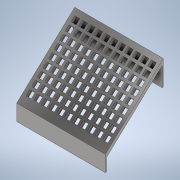
# Autodesk Inventor part: Rejilla_8x8mm
Saved by Autodesk Inventor 2021 (Build 250183000, 183)
## iProperties
Created: 2021-06-27
Part Number: Rejilla_8x8mm
Material: Acero inoxidable
Document SubType Name: Modeling
Designer: artur
Density: 8 g/cm^3
Appearance: Acero - Pulido
Mass: 548.788 g
Surface Area: 547.573 cm^2
Volume: 68.5985 cm^3
Author: artur
Autodesk Inventor part; units mm, degrees
ref_plane "YZ Plane" through (0, 0, 0) normal (1, 0, 0) x (0, 1, 0)
ref_plane "XZ Plane" through (0, 0, 0) normal (0, 1, 0) x (-1, 0, 0)
ref_plane "XY Plane" through (0, 0, 0) normal (0, 0, 1) x (1, 0, 0)
sketch "Boceto7" plane through (-46.053, -27.9809, 0) normal (0, 0, 1) x (1, 0, 0)
  line L0 (118.929, 0) -> (171.1141, 0) construction
  line L1 (-1.0005, -0.9307) -> (-79.0081, -0.9307) construction
  line L2 (-1.0005, -0.9307) -> (89.9995, 83.721)
  line L3 (-1.0005, -0.9307) -> (-1.0005, -25.8991)
  line L4 (-1.0005, -25.8991) -> (0.9995, -25.8991)
  line L5 (0.9995, -25.8991) -> (0.9995, -5.8991)
  line L6 (80.5422, 57.5078) -> (86.2007, 57.5078)
  line L7 (89.9995, 83.721) -> (89.9995, 45.0316)
  line L8 (89.9995, 45.0316) -> (87.9995, 45.0316)
  line L9 (87.9995, 45.0316) -> (87.9995, 75.0316)
  line L10 (0.9995, -5.8991) -> (87.9995, 75.0316)
  dimension "d92" = 137.07
  dimension "d89" = 2
  dimension "d88" = 5
  dimension "d87" = 30
  dimension "d85" = 2
  dimension "d91" = 5
  dimension "d90" = 20
  dimension "d124" = 89
  constraints: 22 end point, 4 horizontal, 2 perpendicular, 2 vertical
  measures "d92" angle of L1 L2
  measures "d89" distance between parallel lines of L5 L3
  measures "d88" distance from line of L2 L9.end
  measures "d87" distance of L8.end L9.end
  measures "d85" distance between parallel lines of L7 L9
  measures "d91" distance from line of L2 L5.end
  measures "d90" distance of L4.end L5.end
  measures "d124" distance between parallel lines of L3 L9
extrude "Extrusión5" add sketch "Boceto7" along normal blind 139
sketch "Boceto8" plane through (-47.0535, -28.9116, 0) normal (-0.6811, 0.7322, 0) x (0, 0, 1)
  line L0 (6, 108.2856) -> (14, 108.2856)
  line L1 (14, 108.2856) -> (14, 116.2856)
  line L2 (14, 116.2856) -> (6, 116.2856)
  line L3 (6, 116.2856) -> (6, 108.2856)
  line L4 (0, 124.2856) -> (139, 124.2856) projected
  line L5 (0, 124.2856) -> (0, 0) projected
  line L6 (18, 108.2856) -> (26, 108.2856)
  line L7 (26, 108.2856) -> (26, 116.2856)
  line L8 (26, 116.2856) -> (18, 116.2856)
  line L9 (18, 116.2856) -> (18, 108.2856)
  line L10 (30, 108.2856) -> (38, 108.2856)
  line L11 (38, 108.2856) -> (38, 116.2856)
  line L12 (38, 116.2856) -> (30, 116.2856)
  line L13 (30, 116.2856) -> (30, 108.2856)
  line L14 (42, 108.2856) -> (50, 108.2856)
  line L15 (50, 108.2856) -> (50, 116.2856)
  line L16 (50, 116.2856) -> (42, 116.2856)
  line L17 (42, 116.2856) -> (42, 108.2856)
  line L18 (54, 108.2856) -> (62, 108.2856)
  line L19 (62, 108.2856) -> (62, 116.2856)
  line L20 (62, 116.2856) -> (54, 116.2856)
  line L21 (54, 116.2856) -> (54, 108.2856)
  line L22 (66, 108.2856) -> (74, 108.2856)
  line L23 (74, 108.2856) -> (74, 116.2856)
  line L24 (74, 116.2856) -> (66, 116.2856)
  line L25 (66, 116.2856) -> (66, 108.2856)
  line L26 (78, 108.2856) -> (86, 108.2856)
  line L27 (86, 108.2856) -> (86, 116.2856)
  line L28 (86, 116.2856) -> (78, 116.2856)
  line L29 (78, 116.2856) -> (78, 108.2856)
  line L30 (90, 108.2856) -> (98, 108.2856)
  line L31 (98, 108.2856) -> (98, 116.2856)
  line L32 (98, 116.2856) -> (90, 116.2856)
  line L33 (90, 116.2856) -> (90, 108.2856)
  line L34 (102, 108.2856) -> (110, 108.2856)
  line L35 (110, 108.2856) -> (110, 116.2856)
  line L36 (110, 116.2856) -> (102, 116.2856)
  line L37 (102, 116.2856) -> (102, 108.2856)
  line L38 (114, 108.2856) -> (122, 108.2856)
  line L39 (122, 108.2856) -> (122, 116.2856)
  line L40 (122, 116.2856) -> (114, 116.2856)
  line L41 (114, 116.2856) -> (114, 108.2856)
  line L42 (126, 108.2856) -> (134, 108.2856)
  line L43 (134, 108.2856) -> (134, 116.2856)
  line L44 (134, 116.2856) -> (126, 116.2856)
  line L45 (126, 116.2856) -> (126, 108.2856)
  line L46 (6, 96.2856) -> (14, 96.2856)
  line L47 (14, 96.2856) -> (14, 104.2856)
  line L48 (14, 104.2856) -> (6, 104.2856)
  line L49 (6, 104.2856) -> (6, 96.2856)
  line L50 (26, 96.2856) -> (26, 104.2856)
  line L51 (18, 96.2856) -> (26, 96.2856)
  line L52 (26, 104.2856) -> (18, 104.2856)
  line L53 (18, 104.2856) -> (18, 96.2856)
  line L54 (30, 104.2856) -> (30, 96.2856)
  line L55 (30, 96.2856) -> (38, 96.2856)
  line L56 (38, 96.2856) -> (38, 104.2856)
  line L57 (42, 104.2856) -> (42, 96.2856)
  line L58 (50, 96.2856) -> (50, 104.2856)
  line L59 (42, 96.2856) -> (50, 96.2856)
  line L60 (50, 104.2856) -> (42, 104.2856)
  line L61 (54, 104.2856) -> (54, 96.2856)
  line L62 (62, 96.2856) -> (62, 104.2856)
  line L63 (54, 96.2856) -> (62, 96.2856)
  line L64 (62, 104.2856) -> (54, 104.2856)
  line L65 (38, 104.2856) -> (30, 104.2856)
  line L66 (90, 104.2856) -> (90, 96.2856)
  line L67 (98, 96.2856) -> (98, 104.2856)
  line L68 (90, 96.2856) -> (98, 96.2856)
  line L69 (102, 104.2856) -> (102, 96.2856)
  line L70 (102, 96.2856) -> (110, 96.2856)
  line L71 (110, 104.2856) -> (102, 104.2856)
  line L72 (98, 104.2856) -> (90, 104.2856)
  line L73 (110, 96.2856) -> (110, 104.2856)
  line L74 (114, 104.2856) -> (114, 96.2856)
  line L75 (114, 96.2856) -> (122, 96.2856)
  line L76 (122, 104.2856) -> (114, 104.2856)
  line L77 (122, 96.2856) -> (122, 104.2856)
  line L78 (126, 104.2856) -> (126, 96.2856)
  line L79 (126, 96.2856) -> (134, 96.2856)
  line L80 (134, 96.2856) -> (134, 104.2856)
  line L81 (134, 104.2856) -> (126, 104.2856)
  line L82 (66, 104.2856) -> (66, 96.2856)
  line L83 (66, 96.2856) -> (74, 96.2856)
  line L84 (74, 104.2856) -> (66, 104.2856)
  line L85 (74, 96.2856) -> (74, 104.2856)
  line L86 (78, 104.2856) -> (78, 96.2856)
  line L87 (78, 96.2856) -> (86, 96.2856)
  line L88 (86, 104.2856) -> (78, 104.2856)
  line L89 (86, 96.2856) -> (86, 104.2856)
  line L90 (6, 84.2856) -> (14, 84.2856)
  line L91 (14, 84.2856) -> (14, 92.2856)
  line L92 (14, 92.2856) -> (6, 92.2856)
  line L93 (6, 92.2856) -> (6, 84.2856)
  line L94 (26, 84.2856) -> (26, 92.2856)
  line L95 (18, 84.2856) -> (26, 84.2856)
  line L96 (26, 92.2856) -> (18, 92.2856)
  line L97 (18, 92.2856) -> (18, 84.2856)
  line L98 (30, 92.2856) -> (30, 84.2856)
  line L99 (30, 84.2856) -> (38, 84.2856)
  line L100 (38, 84.2856) -> (38, 92.2856)
  line L101 (42, 92.2856) -> (42, 84.2856)
  line L102 (50, 84.2856) -> (50, 92.2856)
  line L103 (42, 84.2856) -> (50, 84.2856)
  line L104 (50, 92.2856) -> (42, 92.2856)
  line L105 (54, 92.2856) -> (54, 84.2856)
  line L106 (62, 84.2856) -> (62, 92.2856)
  line L107 (54, 84.2856) -> (62, 84.2856)
  line L108 (62, 92.2856) -> (54, 92.2856)
  line L109 (38, 92.2856) -> (30, 92.2856)
  line L110 (90, 92.2856) -> (90, 84.2856)
  line L111 (98, 84.2856) -> (98, 92.2856)
  line L112 (90, 84.2856) -> (98, 84.2856)
  line L113 (102, 92.2856) -> (102, 84.2856)
  line L114 (102, 84.2856) -> (110, 84.2856)
  line L115 (110, 92.2856) -> (102, 92.2856)
  line L116 (98, 92.2856) -> (90, 92.2856)
  line L117 (110, 84.2856) -> (110, 92.2856)
  line L118 (114, 92.2856) -> (114, 84.2856)
  line L119 (114, 84.2856) -> (122, 84.2856)
  line L120 (122, 92.2856) -> (114, 92.2856)
  line L121 (122, 84.2856) -> (122, 92.2856)
  line L122 (126, 92.2856) -> (126, 84.2856)
  line L123 (126, 84.2856) -> (134, 84.2856)
  line L124 (134, 84.2856) -> (134, 92.2856)
  line L125 (134, 92.2856) -> (126, 92.2856)
  line L126 (66, 92.2856) -> (66, 84.2856)
  line L127 (66, 84.2856) -> (74, 84.2856)
  line L128 (74, 92.2856) -> (66, 92.2856)
  line L129 (74, 84.2856) -> (74, 92.2856)
  line L130 (78, 92.2856) -> (78, 84.2856)
  line L131 (78, 84.2856) -> (86, 84.2856)
  line L132 (86, 92.2856) -> (78, 92.2856)
  line L133 (86, 84.2856) -> (86, 92.2856)
  line L134 (6, 72.2856) -> (14, 72.2856)
  line L135 (14, 72.2856) -> (14, 80.2856)
  line L136 (14, 80.2856) -> (6, 80.2856)
  line L137 (6, 80.2856) -> (6, 72.2856)
  line L138 (26, 72.2856) -> (26, 80.2856)
  line L139 (18, 72.2856) -> (26, 72.2856)
  line L140 (26, 80.2856) -> (18, 80.2856)
  line L141 (18, 80.2856) -> (18, 72.2856)
  line L142 (30, 80.2856) -> (30, 72.2856)
  line L143 (30, 72.2856) -> (38, 72.2856)
  line L144 (38, 72.2856) -> (38, 80.2856)
  line L145 (42, 80.2856) -> (42, 72.2856)
  line L146 (50, 72.2856) -> (50, 80.2856)
  line L147 (42, 72.2856) -> (50, 72.2856)
  line L148 (50, 80.2856) -> (42, 80.2856)
  line L149 (54, 80.2856) -> (54, 72.2856)
  line L150 (62, 72.2856) -> (62, 80.2856)
  line L151 (54, 72.2856) -> (62, 72.2856)
  line L152 (62, 80.2856) -> (54, 80.2856)
  line L153 (38, 80.2856) -> (30, 80.2856)
  line L154 (90, 80.2856) -> (90, 72.2856)
  line L155 (98, 72.2856) -> (98, 80.2856)
  line L156 (90, 72.2856) -> (98, 72.2856)
  line L157 (102, 80.2856) -> (102, 72.2856)
  line L158 (102, 72.2856) -> (110, 72.2856)
  line L159 (110, 80.2856) -> (102, 80.2856)
  line L160 (98, 80.2856) -> (90, 80.2856)
  line L161 (110, 72.2856) -> (110, 80.2856)
  line L162 (114, 80.2856) -> (114, 72.2856)
  line L163 (114, 72.2856) -> (122, 72.2856)
  line L164 (122, 80.2856) -> (114, 80.2856)
  line L165 (122, 72.2856) -> (122, 80.2856)
  line L166 (126, 80.2856) -> (126, 72.2856)
  line L167 (126, 72.2856) -> (134, 72.2856)
  line L168 (134, 72.2856) -> (134, 80.2856)
  line L169 (134, 80.2856) -> (126, 80.2856)
  line L170 (66, 80.2856) -> (66, 72.2856)
  line L171 (66, 72.2856) -> (74, 72.2856)
  line L172 (74, 80.2856) -> (66, 80.2856)
  line L173 (74, 72.2856) -> (74, 80.2856)
  line L174 (78, 80.2856) -> (78, 72.2856)
  line L175 (78, 72.2856) -> (86, 72.2856)
  line L176 (86, 80.2856) -> (78, 80.2856)
  line L177 (86, 72.2856) -> (86, 80.2856)
  line L178 (6, 60.2856) -> (14, 60.2856)
  line L179 (14, 60.2856) -> (14, 68.2856)
  line L180 (14, 68.2856) -> (6, 68.2856)
  line L181 (6, 68.2856) -> (6, 60.2856)
  line L182 (26, 60.2856) -> (26, 68.2856)
  line L183 (18, 60.2856) -> (26, 60.2856)
  line L184 (26, 68.2856) -> (18, 68.2856)
  line L185 (18, 68.2856) -> (18, 60.2856)
  line L186 (30, 68.2856) -> (30, 60.2856)
  line L187 (30, 60.2856) -> (38, 60.2856)
  line L188 (38, 60.2856) -> (38, 68.2856)
  line L189 (42, 68.2856) -> (42, 60.2856)
  line L190 (50, 60.2856) -> (50, 68.2856)
  line L191 (42, 60.2856) -> (50, 60.2856)
  line L192 (50, 68.2856) -> (42, 68.2856)
  line L193 (54, 68.2856) -> (54, 60.2856)
  line L194 (62, 60.2856) -> (62, 68.2856)
  line L195 (54, 60.2856) -> (62, 60.2856)
  line L196 (62, 68.2856) -> (54, 68.2856)
  line L197 (38, 68.2856) -> (30, 68.2856)
  line L198 (90, 68.2856) -> (90, 60.2856)
  line L199 (98, 60.2856) -> (98, 68.2856)
  line L200 (90, 60.2856) -> (98, 60.2856)
  line L201 (102, 68.2856) -> (102, 60.2856)
  line L202 (102, 60.2856) -> (110, 60.2856)
  line L203 (110, 68.2856) -> (102, 68.2856)
  line L204 (98, 68.2856) -> (90, 68.2856)
  line L205 (110, 60.2856) -> (110, 68.2856)
  line L206 (114, 68.2856) -> (114, 60.2856)
  line L207 (114, 60.2856) -> (122, 60.2856)
  line L208 (122, 68.2856) -> (114, 68.2856)
  line L209 (122, 60.2856) -> (122, 68.2856)
  line L210 (126, 68.2856) -> (126, 60.2856)
  line L211 (126, 60.2856) -> (134, 60.2856)
  line L212 (134, 60.2856) -> (134, 68.2856)
  line L213 (134, 68.2856) -> (126, 68.2856)
  line L214 (66, 68.2856) -> (66, 60.2856)
  line L215 (66, 60.2856) -> (74, 60.2856)
  line L216 (74, 68.2856) -> (66, 68.2856)
  line L217 (74, 60.2856) -> (74, 68.2856)
  line L218 (78, 68.2856) -> (78, 60.2856)
  line L219 (78, 60.2856) -> (86, 60.2856)
  line L220 (86, 68.2856) -> (78, 68.2856)
  line L221 (86, 60.2856) -> (86, 68.2856)
  line L222 (6, 48.2856) -> (14, 48.2856)
  line L223 (14, 48.2856) -> (14, 56.2856)
  line L224 (14, 56.2856) -> (6, 56.2856)
  line L225 (6, 56.2856) -> (6, 48.2856)
  line L226 (26, 48.2856) -> (26, 56.2856)
  line L227 (18, 48.2856) -> (26, 48.2856)
  line L228 (26, 56.2856) -> (18, 56.2856)
  line L229 (18, 56.2856) -> (18, 48.2856)
  line L230 (30, 56.2856) -> (30, 48.2856)
  line L231 (30, 48.2856) -> (38, 48.2856)
  line L232 (38, 48.2856) -> (38, 56.2856)
  line L233 (42, 56.2856) -> (42, 48.2856)
  line L234 (50, 48.2856) -> (50, 56.2856)
  line L235 (42, 48.2856) -> (50, 48.2856)
  line L236 (50, 56.2856) -> (42, 56.2856)
  line L237 (54, 56.2856) -> (54, 48.2856)
  line L238 (62, 48.2856) -> (62, 56.2856)
  line L239 (54, 48.2856) -> (62, 48.2856)
  line L240 (62, 56.2856) -> (54, 56.2856)
  line L241 (38, 56.2856) -> (30, 56.2856)
  line L242 (90, 56.2856) -> (90, 48.2856)
  line L243 (98, 48.2856) -> (98, 56.2856)
  line L244 (90, 48.2856) -> (98, 48.2856)
  line L245 (102, 56.2856) -> (102, 48.2856)
  line L246 (102, 48.2856) -> (110, 48.2856)
  line L247 (110, 56.2856) -> (102, 56.2856)
  line L248 (98, 56.2856) -> (90, 56.2856)
  line L249 (110, 48.2856) -> (110, 56.2856)
  line L250 (114, 56.2856) -> (114, 48.2856)
  line L251 (114, 48.2856) -> (122, 48.2856)
  line L252 (122, 56.2856) -> (114, 56.2856)
  line L253 (122, 48.2856) -> (122, 56.2856)
  line L254 (126, 56.2856) -> (126, 48.2856)
  line L255 (126, 48.2856) -> (134, 48.2856)
  line L256 (134, 48.2856) -> (134, 56.2856)
  line L257 (134, 56.2856) -> (126, 56.2856)
  line L258 (66, 56.2856) -> (66, 48.2856)
  line L259 (66, 48.2856) -> (74, 48.2856)
  line L260 (74, 56.2856) -> (66, 56.2856)
  line L261 (74, 48.2856) -> (74, 56.2856)
  line L262 (78, 56.2856) -> (78, 48.2856)
  line L263 (78, 48.2856) -> (86, 48.2856)
  line L264 (86, 56.2856) -> (78, 56.2856)
  line L265 (86, 48.2856) -> (86, 56.2856)
  line L266 (6, 36.2856) -> (14, 36.2856)
  line L267 (14, 36.2856) -> (14, 44.2856)
  line L268 (14, 44.2856) -> (6, 44.2856)
  line L269 (6, 44.2856) -> (6, 36.2856)
  line L270 (26, 36.2856) -> (26, 44.2856)
  line L271 (18, 36.2856) -> (26, 36.2856)
  line L272 (26, 44.2856) -> (18, 44.2856)
  line L273 (18, 44.2856) -> (18, 36.2856)
  line L274 (30, 44.2856) -> (30, 36.2856)
  line L275 (30, 36.2856) -> (38, 36.2856)
  line L276 (38, 36.2856) -> (38, 44.2856)
  line L277 (42, 44.2856) -> (42, 36.2856)
  line L278 (50, 36.2856) -> (50, 44.2856)
  line L279 (42, 36.2856) -> (50, 36.2856)
  line L280 (50, 44.2856) -> (42, 44.2856)
  line L281 (54, 44.2856) -> (54, 36.2856)
  line L282 (62, 36.2856) -> (62, 44.2856)
  line L283 (54, 36.2856) -> (62, 36.2856)
  line L284 (62, 44.2856) -> (54, 44.2856)
  line L285 (38, 44.2856) -> (30, 44.2856)
  line L286 (90, 44.2856) -> (90, 36.2856)
  line L287 (98, 36.2856) -> (98, 44.2856)
  line L288 (90, 36.2856) -> (98, 36.2856)
  line L289 (102, 44.2856) -> (102, 36.2856)
  line L290 (102, 36.2856) -> (110, 36.2856)
  line L291 (110, 44.2856) -> (102, 44.2856)
  line L292 (98, 44.2856) -> (90, 44.2856)
  line L293 (110, 36.2856) -> (110, 44.2856)
  line L294 (114, 44.2856) -> (114, 36.2856)
  line L295 (114, 36.2856) -> (122, 36.2856)
  line L296 (122, 44.2856) -> (114, 44.2856)
  line L297 (122, 36.2856) -> (122, 44.2856)
  line L298 (126, 44.2856) -> (126, 36.2856)
  line L299 (126, 36.2856) -> (134, 36.2856)
  line L300 (134, 36.2856) -> (134, 44.2856)
  line L301 (134, 44.2856) -> (126, 44.2856)
  line L302 (66, 44.2856) -> (66, 36.2856)
  line L303 (66, 36.2856) -> (74, 36.2856)
  line L304 (74, 44.2856) -> (66, 44.2856)
  line L305 (74, 36.2856) -> (74, 44.2856)
  line L306 (78, 44.2856) -> (78, 36.2856)
  line L307 (78, 36.2856) -> (86, 36.2856)
  line L308 (86, 44.2856) -> (78, 44.2856)
  line L309 (86, 36.2856) -> (86, 44.2856)
  line L310 (6, 24.2856) -> (14, 24.2856)
  line L311 (14, 24.2856) -> (14, 32.2856)
  line L312 (14, 32.2856) -> (6, 32.2856)
  line L313 (6, 32.2856) -> (6, 24.2856)
  line L314 (26, 24.2856) -> (26, 32.2856)
  line L315 (18, 24.2856) -> (26, 24.2856)
  line L316 (26, 32.2856) -> (18, 32.2856)
  line L317 (18, 32.2856) -> (18, 24.2856)
  line L318 (30, 32.2856) -> (30, 24.2856)
  line L319 (30, 24.2856) -> (38, 24.2856)
  line L320 (38, 24.2856) -> (38, 32.2856)
  line L321 (42, 32.2856) -> (42, 24.2856)
  line L322 (50, 24.2856) -> (50, 32.2856)
  line L323 (42, 24.2856) -> (50, 24.2856)
  line L324 (50, 32.2856) -> (42, 32.2856)
  line L325 (54, 32.2856) -> (54, 24.2856)
  line L326 (62, 24.2856) -> (62, 32.2856)
  line L327 (54, 24.2856) -> (62, 24.2856)
  line L328 (62, 32.2856) -> (54, 32.2856)
  line L329 (38, 32.2856) -> (30, 32.2856)
  line L330 (90, 32.2856) -> (90, 24.2856)
  line L331 (98, 24.2856) -> (98, 32.2856)
  line L332 (90, 24.2856) -> (98, 24.2856)
  line L333 (102, 32.2856) -> (102, 24.2856)
  line L334 (102, 24.2856) -> (110, 24.2856)
  line L335 (110, 32.2856) -> (102, 32.2856)
  line L336 (98, 32.2856) -> (90, 32.2856)
  line L337 (110, 24.2856) -> (110, 32.2856)
  line L338 (114, 32.2856) -> (114, 24.2856)
  line L339 (114, 24.2856) -> (122, 24.2856)
  line L340 (122, 32.2856) -> (114, 32.2856)
  line L341 (122, 24.2856) -> (122, 32.2856)
  line L342 (126, 32.2856) -> (126, 24.2856)
  line L343 (126, 24.2856) -> (134, 24.2856)
  line L344 (134, 24.2856) -> (134, 32.2856)
  line L345 (134, 32.2856) -> (126, 32.2856)
  line L346 (66, 32.2856) -> (66, 24.2856)
  line L347 (66, 24.2856) -> (74, 24.2856)
  line L348 (74, 32.2856) -> (66, 32.2856)
  line L349 (74, 24.2856) -> (74, 32.2856)
  line L350 (78, 32.2856) -> (78, 24.2856)
  line L351 (78, 24.2856) -> (86, 24.2856)
  line L352 (86, 32.2856) -> (78, 32.2856)
  line L353 (86, 24.2856) -> (86, 32.2856)
  line L354 (6, 12.2856) -> (14, 12.2856)
  line L355 (14, 12.2856) -> (14, 20.2856)
  line L356 (14, 20.2856) -> (6, 20.2856)
  line L357 (6, 20.2856) -> (6, 12.2856)
  line L358 (26, 12.2856) -> (26, 20.2856)
  line L359 (18, 12.2856) -> (26, 12.2856)
  line L360 (26, 20.2856) -> (18, 20.2856)
  line L361 (18, 20.2856) -> (18, 12.2856)
  line L362 (30, 20.2856) -> (30, 12.2856)
  line L363 (30, 12.2856) -> (38, 12.2856)
  line L364 (38, 12.2856) -> (38, 20.2856)
  line L365 (42, 20.2856) -> (42, 12.2856)
  line L366 (50, 12.2856) -> (50, 20.2856)
  line L367 (42, 12.2856) -> (50, 12.2856)
  line L368 (50, 20.2856) -> (42, 20.2856)
  line L369 (54, 20.2856) -> (54, 12.2856)
  line L370 (62, 12.2856) -> (62, 20.2856)
  line L371 (54, 12.2856) -> (62, 12.2856)
  line L372 (62, 20.2856) -> (54, 20.2856)
  line L373 (38, 20.2856) -> (30, 20.2856)
  line L374 (90, 20.2856) -> (90, 12.2856)
  line L375 (98, 12.2856) -> (98, 20.2856)
  line L376 (90, 12.2856) -> (98, 12.2856)
  line L377 (102, 20.2856) -> (102, 12.2856)
  line L378 (102, 12.2856) -> (110, 12.2856)
  line L379 (110, 20.2856) -> (102, 20.2856)
  line L380 (98, 20.2856) -> (90, 20.2856)
  line L381 (110, 12.2856) -> (110, 20.2856)
  line L382 (114, 20.2856) -> (114, 12.2856)
  line L383 (114, 12.2856) -> (122, 12.2856)
  line L384 (122, 20.2856) -> (114, 20.2856)
  line L385 (122, 12.2856) -> (122, 20.2856)
  line L386 (126, 20.2856) -> (126, 12.2856)
  line L387 (126, 12.2856) -> (134, 12.2856)
  line L388 (134, 12.2856) -> (134, 20.2856)
  line L389 (134, 20.2856) -> (126, 20.2856)
  line L390 (66, 20.2856) -> (66, 12.2856)
  line L391 (66, 12.2856) -> (74, 12.2856)
  line L392 (74, 20.2856) -> (66, 20.2856)
  line L393 (74, 12.2856) -> (74, 20.2856)
  line L394 (78, 20.2856) -> (78, 12.2856)
  line L395 (78, 12.2856) -> (86, 12.2856)
  line L396 (86, 20.2856) -> (78, 20.2856)
  line L397 (86, 12.2856) -> (86, 20.2856)
  dimension "d111" = 8
  dimension "d110" = 8
  dimension "d109" = 8
  dimension "d103" = 12
  dimension "d117" = 12
  dimension "d122" = 6
  constraints: 792 end point, 2 horizontal, 2 parallel, 1 perpendicular, 1 vertical, 784 other
  measures "d111" distance of L0.end L1.end
  measures "d110" distance of L0.start L0.end
  measures "d109" distance between parallel lines of L4 L2
  measures "d103" distance of L0.start L6.start
  measures "d117" distance of L0.start L46.start
  measures "d122" distance between parallel lines of L5 L3
extrude "Extrusión6" cut sketch "Boceto8" against normal up to surface (5 mm away)
